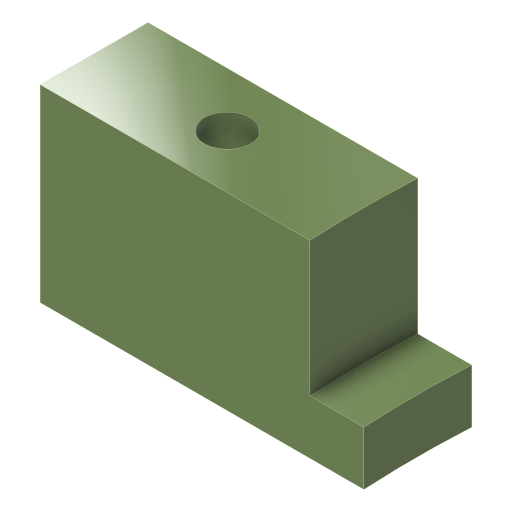
# Autodesk Inventor part: holder
Saved by Autodesk Inventor 2024.2 (Build 282272000, 272)
## iProperties
Created: 2023-12-04
Part Number: holder
Material: Generic
Document SubType Name: Modeling
Designer: kuzmin
Density: 1 g/cm^3
Appearance: Dark Olive
Author: kuzmin
Autodesk Inventor part; units mm, degrees
ref_plane "YZ Plane" through (0, 0, 0) normal (1, 0, 0) x (0, 1, 0)
ref_plane "XZ Plane" through (0, 0, 0) normal (0, 1, 0) x (-1, 0, 0)
ref_plane "XY Plane" through (0, 0, 0) normal (0, 0, 1) x (1, 0, 0)
sketch "Sketch1" plane through (0, 0, 0) normal (0, 0, 1) x (1, 0, 0)
  arc A0 (-4, 0.1053) -> (4, 0.1053) centre (0, 76) ccw
  line L0 (4, 0.1053) -> (4, -19.8947)
  line L1 (4, -19.8947) -> (-4, -19.8947)
  line L2 (-4, -19.8947) -> (-4, 0.1053)
  arc A1 (-4, 4.1112) -> (4, 4.1112) centre (0, 76) ccw
  line L3 (4, 0.1053) -> (4, 4.1112)
  line L4 (-4, 0.1053) -> (-4, 4.1112)
  point P0 (0, 0)
  point P1 (0, -19.8947)
  point P2 (0, 0)
  dimension "d0" = 76
  dimension "d1" = 4
  dimension "d2" = 8
  dimension "d3" = 20
  constraints: 10 end point, 6 point on circle, 3 vertical, 2 centre point, 2 coincident, 2 perpendicular, 2 vertical alignment, 1 midpoint
  measures "d0" radius of A0
  measures "d1" radial gap between concentric circles of A0 A1
  measures "d2" distance of L0.end L1.end
  measures "d3" distance of L1.end L2.end
extrude "Extrusion1" add sketch "Sketch1" along normal blind 14 contours A0 L0 L1 L2
extrude "Extrusion2" add sketch "Sketch1" along normal blind 4 contours L4 A1 L3 A0
sketch "Sketch2" plane through (0, 0, 14) normal (0, 0, 1) x (1, 0, 0)
  circle A0 centre (0, -10) radius 1.7
  arc A1 (-4, 0.1053) -> (4, 0.1053) centre (0, 76) ccw projected
  point P0 (0, 0)
  point P1 (0, 0)
  dimension "d11" = 0
  dimension "d8" = 3.4
  dimension "d9" = 10
  constraints: 1 centre point, 1 point on circle
  measures "d8" diameter of A0
  measures "d9" distance of A0.centre point (0, 0)
extrude "Extrusion3" cut sketch "Sketch2" against normal through all
body "Solid1"
